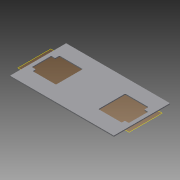
# Autodesk Inventor part: base robot
Saved by Autodesk Inventor 2016 (Build 200138000, 138)
## iProperties
Created: 2012-11-07
Part Number: base robot
Material: Générique
Document SubType Name: Modeling
Designer: Aegir
Density: 1 g/cm^3
Appearance: Par défaut
Author: Aegir
Autodesk Inventor part; units mm, degrees
ref_plane "YZ Plane" through (0, 0, 0) normal (1, 0, 0) x (0, 1, 0)
ref_plane "XZ Plane" through (0, 0, 0) normal (0, 1, 0) x (-1, 0, 0)
ref_plane "XY Plane" through (0, 0, 0) normal (0, 0, 1) x (1, 0, 0)
ref_plane "Plan de construction1" through (0, 0, 0) normal (0, 0, 1) x (1, 0, 0)
sketch "Esquisse1" plane through (0, 0, 0) normal (0, 0, 1) x (1, 0, 0)
  line L0 (-259.3709, 57.007) -> (-192, 57.007)
  line L1 (-190, 55.007) -> (-190, -23.1037)
  line L2 (-192, -25.1037) -> (-259.3709, -25.1037)
  line L3 (-263.3709, 43.802) -> (-271.3754, 43.802)
  line L4 (-273.3754, 41.802) -> (-273.3754, -13.5001)
  line L5 (-271.3754, -15.5001) -> (-263.3709, -15.5001)
  line L6 (-261.3709, -23.1037) -> (-261.3709, -17.5001)
  line L7 (-261.3709, 45.802) -> (-261.3709, 55.007)
  arc A0 (-263.3709, 43.802) -> (-261.3709, 45.802) centre (-263.3709, 45.802) ccw
  arc A1 (-190, 55.007) -> (-192, 57.007) centre (-192, 55.007) ccw
  arc A2 (-192, -25.1037) -> (-190, -23.1037) centre (-192, -23.1037) ccw
  arc A3 (-261.3709, -17.5001) -> (-263.3709, -15.5001) centre (-263.3709, -17.5001) ccw
  arc A4 (-261.3709, -23.1037) -> (-259.3709, -25.1037) centre (-259.3709, -23.1037) ccw
  arc A5 (-273.3754, -13.5001) -> (-271.3754, -15.5001) centre (-271.3754, -13.5001) ccw
  arc A6 (-271.3754, 43.802) -> (-273.3754, 41.802) centre (-271.3754, 41.802) ccw
  arc A7 (-259.3709, 57.007) -> (-261.3709, 55.007) centre (-259.3709, 55.007) ccw
  line L8 (-190, 25.8053) -> (-162, 25.8053) projected
  line L9 (-125, 120.1339) -> (-125, -94.4398)
  line L10 (-280, 60.1339) -> (30, 60.1339) projected
  line L11 (30, 60.1339) -> (30, -31.8661) projected
  line L12 (9.3709, 57.007) -> (-58, 57.007)
  line L13 (-60, 55.007) -> (-60, -23.1037)
  line L14 (-58, -25.1037) -> (9.3709, -25.1037)
  line L15 (13.3709, 43.802) -> (21.3754, 43.802)
  line L16 (23.3754, 41.802) -> (23.3754, -13.5001)
  line L17 (21.3754, -15.5001) -> (13.3709, -15.5001)
  line L18 (11.3709, -23.1037) -> (11.3709, -17.5001)
  line L19 (11.3709, 45.802) -> (11.3709, 55.007)
  arc A8 (11.3709, 45.802) -> (13.3709, 43.802) centre (13.3709, 45.802) ccw
  arc A9 (-58, 57.007) -> (-60, 55.007) centre (-58, 55.007) ccw
  arc A10 (-60, -23.1037) -> (-58, -25.1037) centre (-58, -23.1037) ccw
  arc A11 (13.3709, -15.5001) -> (11.3709, -17.5001) centre (13.3709, -17.5001) ccw
  arc A12 (9.3709, -25.1037) -> (11.3709, -23.1037) centre (9.3709, -23.1037) ccw
  arc A13 (21.3754, -15.5001) -> (23.3754, -13.5001) centre (21.3754, -13.5001) ccw
  arc A14 (23.3754, 41.802) -> (21.3754, 43.802) centre (21.3754, 41.802) ccw
  arc A15 (11.3709, 55.007) -> (9.3709, 57.007) centre (9.3709, 55.007) ccw
  line L20 (-125, 120.1339) -> (-284, 120.1339)
  line L21 (-284, 120.1339) -> (-284, -51.8661)
  line L22 (-284, -51.8661) -> (-125, -51.8661)
  line L23 (-125, -51.8661) -> (-125, 120.1339)
  line L24 (-280, -31.8661) -> (-280, 60.1339) projected
  line L25 (-323.0211, 14.1339) -> (69.534, 14.1339)
  line L26 (-125, 120.1339) -> (34, 120.1339)
  line L27 (34, 120.1339) -> (34, -51.8661)
  line L28 (34, -51.8661) -> (-125, -51.8661)
  point P0 (0, 0)
  dimension "d0" = 2
  dimension "d1" = 155
  dimension "d4" = 4
  dimension "d5" = 172
  dimension "d10" = 20
  constraints: 50 end point, 32 point on circle, 26 symmetric about line, 16 centre point, 16 tangent, 7 equal radius, 6 parallel, 5 perpendicular, 3 horizontal, 1 point on line, 8 other
  measures "d0" radius of A0
  measures "d1" distance between parallel lines of L11 L9
  measures "d4" distance from line of L21 L24.start
  measures "d5" distance of L20.end L21.end
  measures "d10" vertical distance of L21.end L24.start
extrude "Extrusion1" add sketch "Esquisse1" along normal blind 3 contours A7 L7 A0 L3 A6 L4 L25 L24 L10 L9 L1 A1 L0 | L25 L9 L22 L21 L4 A5 L5 A3 L6 A4 L2 A2 L1 | L25 L13 A10 L14 A12 L18 A11 L17 A13 L16 L27 L28 L9 | L9 L10 L11 L25 L16 A14 L15 A8 L19 A15 L12 A9 L13 | L25 L21 L20 L9 L10 L24 | L9 L26 L27 L25 L11 L10
